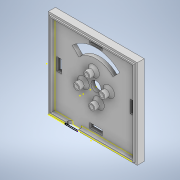
# Autodesk Inventor part: bottomplate
Saved by Autodesk Inventor 2022 (Build 260153000, 153)
## iProperties
Created: 2023-12-05
Part Number: bottomplate
Material: Generisch
Document SubType Name: Modeling
Designer: Marc Panse
Density: 1 g/cm^3
Appearance: Vorgabe
Author: Marc Panse
## iProperties of the stored document bottomplate_3D-Druck.ipt
Created: 2023-12-05
Part Number: bottomplate_3D-Druck
Material: Generisch
Document SubType Name: Modeling
Designer: Marc Panse
Density: 1 g/cm^3
Appearance: Vorgabe
Author: Marc Panse
Autodesk Inventor part; units mm, degrees
ref_plane "YZ Plane" through (0, 0, 0) normal (1, 0, 0) x (0, 1, 0)
ref_plane "XZ Plane" through (0, 0, 0) normal (0, 1, 0) x (-1, 0, 0)
ref_plane "XY Plane" through (0, 0, 0) normal (0, 0, 1) x (1, 0, 0)
sketch "Skizze1" plane through (0, 0, 0) normal (0, 0, 1) x (1, 0, 0)
  line L0 (-33.02, -33.02) -> (33.02, -33.02)
  line L1 (33.02, -33.02) -> (33.02, 33.02)
  line L2 (33.02, 33.02) -> (-33.02, 33.02)
  line L3 (-33.02, 33.02) -> (-33.02, -33.02)
  line L4 (-33.02, -33.02) -> (33.02, 33.02) construction
  line L5 (33.02, -33.02) -> (-33.02, 33.02) construction
  line L6 (-34, -34) -> (34, -34)
  line L7 (34, -34) -> (34, 34)
  line L8 (34, 34) -> (-34, 34)
  line L9 (-34, 34) -> (-34, -34)
  line L10 (-34, -34) -> (34, 34) construction
  line L11 (34, -34) -> (-34, 34) construction
  point P0 (0, 0)
  dimension "d0" = 66.04
  dimension "d1" = 66.04
  dimension "d2" = 68
  dimension "d3" = 68
  constraints: 24 end point, 4 midpoint, 4 parallel, 2 horizontal, 2 perpendicular
  measures "d0" distance of L2.end L1.end
  measures "d1" distance of L1.end L0.end
  measures "d2" distance of L8.end L7.end
  measures "d3" distance of L7.end L6.end
extrude "Extrusion1" add sketch "Skizze1" along normal blind 6.5
sketch "Skizze2" plane through (0, 0, 6.5) normal (0, 0, 1) x (1, 0, 0)
  line L0 (-33.02, 33.02) -> (33.02, 33.02) projected
  line L1 (-33.02, -33.02) -> (33.02, -33.02)
  line L2 (33.02, -33.02) -> (33.02, 33.02)
  line L3 (33.02, 33.02) -> (-33.02, 33.02)
  line L4 (-33.02, 33.02) -> (-33.02, -33.02)
  line L5 (-33.02, -33.02) -> (33.02, 33.02) construction
  line L6 (33.02, -33.02) -> (-33.02, 33.02) construction
  line L7 (34, -34) -> (34, 34) projected
  line L8 (34, 34) -> (-34, 34) projected
  line L9 (-34, 34) -> (-34, -34) projected
  line L10 (-34, -34) -> (34, -34) projected
  line L11 (-33.02, -33.02) -> (-33.02, 33.02) projected
  line L12 (-33.02, 33.02) -> (33.02, 33.02) projected
  line L13 (33.02, 33.02) -> (33.02, -33.02) projected
  line L14 (33.02, -33.02) -> (-33.02, -33.02) projected
  point P0 (0, 0)
  constraints: 12 end point, 2 midpoint, 2 parallel, 1 horizontal, 1 perpendicular
extrude "Extrusion2" add sketch "Skizze2" along normal blind 2 contours L0 L2 L1 L4 | L10 L9 L8 L7
sketch "Skizze3" plane through (0, 0, 6.5) normal (0, 0, -1) x (-1, 0, 0)
  line L0 (-27.94, -27.94) -> (27.94, -27.94)
  line L1 (27.94, -27.94) -> (27.94, 27.94)
  line L2 (27.94, 27.94) -> (-27.94, 27.94)
  line L3 (-27.94, 27.94) -> (-27.94, -27.94)
  line L4 (-27.94, -27.94) -> (27.94, 27.94) construction
  line L5 (27.94, -27.94) -> (-27.94, 27.94) construction
  circle A0 centre (-27.94, 27.94) radius 3.35
  circle A1 centre (27.94, 27.94) radius 3.35
  circle A2 centre (27.94, -27.94) radius 3.35
  circle A3 centre (-27.94, -27.94) radius 3.35
  point P0 (0, 0)
  dimension "d8" = 55.88
  dimension "d9" = 55.88
  dimension "d10" = 6.7
  dimension "d11" = 6.7
  dimension "d12" = 6.7
  dimension "d13" = 6.7
  constraints: 12 end point, 4 centre point, 4 coincident, 2 midpoint, 2 parallel, 1 horizontal, 1 perpendicular
  measures "d8" distance of L2.end L1.end
  measures "d9" distance of L1.end L0.end
  measures "d10" diameter of A0
  measures "d11" diameter of A1
  measures "d12" diameter of A2
  measures "d13" diameter of A3
extrude "Extrusion3" add sketch "Skizze3" along normal blind 5 contours L3 A3 L0 | L0 A3 L3 | A2 L1 L0 | L0 L1 A2 | A0 L2 L3 | L3 L2 A0 | A1 L2 L1 | L1 L2 A1
sketch "Skizze4" plane through (27.94, 27.94, 1.5) normal (0, 0, -1) x (-1, 0, 0)
  circle A0 centre (0, 0) radius 1.1
  circle A1 centre (55.88, 0) radius 3.35 projected
  circle A2 centre (55.88, 0) radius 1.1
  circle A3 centre (55.88, -55.88) radius 3.35 projected
  circle A4 centre (55.88, -55.88) radius 1.1
  circle A5 centre (0, -55.88) radius 3.35 projected
  circle A6 centre (0, -55.88) radius 1.1
  point P0 (27.94, -27.94)
  dimension "d17" = 2.2
  dimension "d18" = 2.2
  dimension "d19" = 2.2
  dimension "d20" = 2.2
  constraints: 4 centre point, 3 coincident
  measures "d17" diameter of A0
  measures "d18" diameter of A2
  measures "d19" diameter of A4
  measures "d20" diameter of A6
extrude "Extrusion4" cut sketch "Skizze4" against normal blind 5 contours A0 | A2 | A4 | A6
sketch "Skizze5" plane through (0, 0, 0) normal (0, 0, -1) x (-1, 0, 0)
  line L0 (-34, -34) -> (-34, 34) projected
  line L1 (34, -34) -> (-34, -34) projected
  line L2 (34, 34) -> (34, -34) projected
  line L3 (-34, 34) -> (34, 34) projected
  line L4 (33.02, -33.02) -> (33.02, 33.02) projected
  line L5 (-33.02, -33.02) -> (33.02, -33.02) projected
  line L6 (-33.02, 33.02) -> (-33.02, -33.02) projected
  line L7 (33.02, 33.02) -> (-33.02, 33.02) projected
  point P0 (0, 0)
extrude "Extrusion5" add sketch "Skizze5" along normal blind 4
sketch "Skizze6" plane through (0, 0, -4) normal (0, 0, -1) x (-1, 0, 0)
  line L0 (-33.02, -33.02) -> (33.02, -33.02)
  line L1 (33.02, -33.02) -> (33.02, 33.02)
  line L2 (33.02, 33.02) -> (-33.02, 33.02)
  line L3 (-33.02, 33.02) -> (-33.02, -33.02)
  line L4 (-33.02, -33.02) -> (33.02, 33.02) construction
  line L5 (33.02, -33.02) -> (-33.02, 33.02) construction
  line L6 (33.02, -33.02) -> (20.02, -33.02)
  line L7 (-33.02, -33.02) -> (33.02, -33.02) projected
  line L8 (20.02, -33.02) -> (10.08, -33.02)
  line L9 (34, -34) -> (-34, -34) projected
  line L10 (10.08, -33.02) -> (20.02, -33.02)
  line L11 (20.02, -33.02) -> (20.02, -34)
  line L12 (20.02, -34) -> (10.08, -34)
  line L13 (10.08, -34) -> (10.08, -33.02)
  point P0 (0, 0)
  point P1 (-24.13, -33.02)
  point P2 (24.13, -33.02)
  dimension "d25" = 66.04
  dimension "d26" = 66.04
  dimension "d27" = 13
  dimension "d28" = 9.94
  constraints: 24 end point, 4 parallel, 3 point on line, 2 horizontal, 2 midpoint, 2 perpendicular
  measures "d25" distance of L2.end L1.end
  measures "d26" distance of L1.end L0.end
  measures "d27" distance of L0.end L6.end
  measures "d28" distance of L6.end L8.end
extrude "Extrusion6" cut sketch "Skizze6" against normal blind 4 contours L0 L11 L9 L13
fillet "Rundung2" radius 1.75 2 edges at (-10.08, -33.51, 0) (-20.02, -33.51, 0)
sketch "Skizze7" plane through (0, 0, -4) normal (0, 0, -1) x (-1, 0, 0)
  line L0 (34, 34) -> (-34, 34) projected
  line L1 (-34, -34) -> (34, -34)
  line L2 (34, -34) -> (34, 34)
  line L3 (34, 34) -> (-34, 34)
  line L4 (-34, 34) -> (-34, -34)
  line L5 (-34, -34) -> (34, 34) construction
  line L6 (34, -34) -> (-34, 34) construction
  line L7 (-35, -35) -> (35, -35)
  line L8 (35, -35) -> (35, 35)
  line L9 (35, 35) -> (-35, 35)
  line L10 (-35, 35) -> (-35, -35)
  line L11 (-35, -35) -> (35, 35) construction
  line L12 (35, -35) -> (-35, 35) construction
  point P0 (0, 0)
  point P1 (-34, 34)
  dimension "d32" = 70
  dimension "d33" = 70
  constraints: 24 end point, 4 midpoint, 4 parallel, 2 horizontal, 2 perpendicular
  measures "d32" distance of L9.end L8.end
  measures "d33" distance of L8.end L7.end
extrude "Extrusion7" add sketch "Skizze7" against normal up to surface (12.5 mm away)
sketch "Skizze8" plane through (-20.02, -34, -4) normal (0, 1, 0) x (1, 0, 0)
  line L0 (9.94, -2.25) -> (9.94, 0) projected
  line L1 (0, 0) -> (9.94, 0) projected
  line L2 (0, 0) -> (0, -2.25) projected
  arc A0 (0, -2.25) -> (1.75, -4) centre (1.75, -2.25) ccw projected
  line L3 (1.75, -4) -> (8.19, -4) projected
  arc A1 (8.19, -4) -> (9.94, -2.25) centre (8.19, -2.25) ccw projected
  point P0 (20.02, -4)
extrude "Extrusion8" cut sketch "Skizze8" against normal blind 10
sketch "Skizze9" plane through (0, 0, -4) normal (0, 0, -1) x (-1, 0, 0)
  line L0 (-33.52, 33.52) -> (33.52, 33.52)
  line L1 (33.52, 33.52) -> (33.52, -33.52)
  line L2 (33.52, -33.52) -> (-33.52, -33.52)
  line L3 (-33.52, -33.52) -> (-33.52, 33.52)
  line L4 (-33.52, 33.52) -> (33.52, -33.52) construction
  line L5 (33.52, 33.52) -> (-33.52, -33.52) construction
  line L6 (10.08, -35) -> (10.08, -33.02) projected
  line L7 (10.08, -33.02) -> (-33.02, -33.02) projected
  line L8 (-33.02, -33.02) -> (-33.02, 33.02) projected
  line L9 (-33.02, 33.02) -> (33.02, 33.02) projected
  line L10 (33.02, 33.02) -> (33.02, -33.02) projected
  line L11 (33.02, -33.02) -> (20.02, -33.02) projected
  line L12 (20.02, -33.02) -> (20.02, -35) projected
  line L13 (20.02, -35) -> (35, -35) projected
  line L14 (35, -35) -> (35, 35) projected
  line L15 (35, 35) -> (-35, 35) projected
  line L16 (-35, 35) -> (-35, -35) projected
  line L17 (-35, -35) -> (10.08, -35) projected
  point P0 (0, 0)
  point P1 (10.08, -33.52)
  point P2 (20.02, -33.52)
  dimension "d38" = 67.04
  dimension "d39" = 67.04
  constraints: 12 end point, 2 midpoint, 2 parallel, 1 horizontal, 1 perpendicular
  measures "d38" distance of L1.end L2.end
  measures "d39" distance of L0.end L1.end
extrude "Extrusion9" cut sketch "Skizze9" against normal up to surface (10.5 mm away) contours L0 L1 L2 L12 L11 L10 L9 L8 L7 L6 L3
fillet "Rundung3" radius 2 4 edges at (31.29, -27.94, 6.5) (31.29, 27.94, 6.5) (-24.59, 27.94, 6.5) (-24.59, -27.94, 6.5)
sketch "Skizze10" plane through (-35, -35, -4) normal (-1, 0, 0) x (0, 0, 1)
  point P0 (4, 35)
sketch "Skizze11" plane through (0, 0, 8.5) normal (0, 0, 1) x (1, 0, 0)
  point P0 (0, 0)
sketch "Skizze12" plane through (-18.27, -33.02, 0) normal (0, 1, 0) x (1, 0, 0)
  line L0 (-1.75, 1.75) -> (-1.75, -6.5) projected
  line L1 (8.19, -6.5) -> (-1.75, -6.5) projected
  line L2 (8.19, -6.5) -> (8.19, 1.75) projected
  arc A0 (6.44, 0) -> (8.19, 1.75) centre (6.44, 1.75) ccw projected
  line L3 (6.44, 0) -> (0, 0) projected
  arc A1 (-1.75, 1.75) -> (0, 0) centre (0, 1.75) ccw projected
  point P0 (18.27, 0)
extrude "Extrusion10" cut sketch "Skizze12" against normal up to surface (0.5 mm away)
sketch "Skizze13" plane through (0, 0, -4) normal (0, 0, -1) x (-1, 0, 0)
  circle A0 centre (0, 0) radius 4
  line L0 (0, 0) -> (-10.0581, 1.7135)
  line L1 (0, 0) -> (10.203, 0) construction
  line L2 (0, 0) -> (1.8539, 9.7483)
  line L3 (0, 0) -> (9.923, 0) construction
  line L4 (0, 0) -> (9.888, -2.1637)
  line L5 (0, 0) -> (10.122, 0) construction
  line L6 (0, 0) -> (-2.0234, -10.1982)
  line L7 (0, 0) -> (10.397, 0) construction
  circle A1 centre (-2.0234, -10.1982) radius 2.5
  circle A2 centre (-10.0581, 1.7135) radius 2.5
  circle A3 centre (1.8539, 9.7483) radius 2.5
  circle A4 centre (9.888, -2.1637) radius 2.5
  dimension "d59" = 8
  dimension "d60" = 10.203
  dimension "d61" = 170.332
  dimension "d62" = 9.923
  dimension "d63" = 79.232
  dimension "d64" = 10.122
  dimension "d65" = 12.343
  dimension "d66" = 10.397
  dimension "d67" = 101.222
  dimension "d68" = 5
  dimension "d69" = 5
  dimension "d70" = 5
  dimension "d71" = 5
  constraints: 16 end point, 5 centre point, 5 coincident, 4 equal length, 4 horizontal
  measures "d59" diameter of A0
  measures "d60" distance of L0.start L0.end
  measures "d61" angle of L1 L0
  measures "d62" distance of L0.start L2.end
  measures "d63" angle of L3 L2
  measures "d64" distance of L0.start L4.end
  measures "d65" angle of L4 L5
  measures "d66" distance of L0.start L6.end
  measures "d67" angle of L6 L7
  measures "d68" diameter of A1
  measures "d69" diameter of A2
  measures "d70" diameter of A3
  measures "d71" diameter of A4
extrude "Extrusion11" add sketch "Skizze13" against normal up to surface (10.5 mm away) contours A1 | A2 | A3 | A4
sketch "Skizze14" plane through (-9.888, -2.1637, -4) normal (0, 0, -1) x (-1, 0, 0)
  circle A0 centre (0, 0) radius 2.5 projected
  circle A1 centre (-11.9114, -8.0345) radius 2.5 projected
  circle A2 centre (-19.9461, 3.8772) radius 2.5 projected
  circle A3 centre (-8.0341, 11.912) radius 2.5 projected
  point P0 (-9.888, 2.1637)
extrude "Extrusion12" cut sketch "Skizze14" against normal blind 5.5
fillet "Rundung4" radius 4 4 edges at (12.5581, 1.7135, 6.5) (0.6461, 9.7483, 6.5) (-7.388, -2.1637, 6.5) (4.5234, -10.1982, 6.5)
sketch "Skizze15" plane through (-9.888, -2.1637, 1.5) normal (0, 0, -1) x (-1, 0, 0)
  circle A0 centre (0, 0) radius 1
  circle A1 centre (-11.9114, -8.0345) radius 2.5 projected
  circle A2 centre (-11.9114, -8.0345) radius 1
  circle A3 centre (-19.9461, 3.8772) radius 2.5 projected
  circle A4 centre (-19.9461, 3.8772) radius 1
  circle A5 centre (-8.0341, 11.912) radius 2.5 projected
  circle A6 centre (-8.0341, 11.912) radius 1
  point P0 (-9.888, 2.1637)
  dimension "d77" = 2
  dimension "d78" = 2
  dimension "d79" = 2
  dimension "d80" = 2
  constraints: 4 centre point, 3 coincident
  measures "d77" diameter of A0
  measures "d78" diameter of A2
  measures "d79" diameter of A4
  measures "d80" diameter of A6
extrude "Extrusion13" cut sketch "Skizze15" against normal blind 5 contours A0 | A2 | A4 | A6
chamfer "Fase1" distance 4 angle 45 4 edges at (-33.52, 0, 6.5) (0, -33.52, 6.5) (0, 33.52, 6.5) (33.52, 0, 6.5)
sketch "Skizze16" plane through (10.0581, 1.7135, 1.5) normal (0, 0, -1) x (-1, 0, 0)
  circle A0 centre (0, 0) radius 1.6
  circle A1 centre (8.0347, -11.9117) radius 1 projected
  circle A2 centre (8.0347, -11.9117) radius 1.6
  circle A3 centre (11.912, 8.0348) radius 1 projected
  circle A4 centre (11.912, 8.0348) radius 1.6
  circle A5 centre (19.9461, -3.8772) radius 1 projected
  circle A6 centre (19.9461, -3.8772) radius 1.6
  point P0 (10.0581, -1.7135)
  dimension "d86" = 3.2
  dimension "d87" = 3.2
  dimension "d88" = 3.2
  dimension "d89" = 3.2
  constraints: 4 centre point, 3 coincident
  measures "d86" diameter of A0
  measures "d87" diameter of A2
  measures "d88" diameter of A4
  measures "d89" diameter of A6
extrude "Extrusion14" cut sketch "Skizze16" against normal blind 10 contours A0 | A1 | A2 | A3 | A4 | A5 | A6
chamfer "Fase2" distance 2 angle 45 4 edges at (-8.288, -2.1637, 8.5) (3.6234, -10.1982, 8.5) (11.6581, 1.7135, 8.5) (-0.2539, 9.7483, 8.5)
sketch "Skizze17" plane through (0, 0, 8.5) normal (0, 0, 1) x (1, 0, 0)
  circle A0 centre (10.0581, 1.7135) radius 3.6 projected
  circle A1 centre (-9.888, -2.1637) radius 3.6 projected
  line L0 (35, 35) -> (-35, 35) projected
  line L1 (-35, 35) -> (-35, -35) projected
  line L2 (-35, -35) -> (35, -35) projected
  line L3 (35, -35) -> (35, 35) projected
  circle A2 centre (2.0234, -10.1982) radius 3.6 projected
  circle A3 centre (-1.8539, 9.7483) radius 3.6 projected
  line L4 (-35, -35) -> (35, -35) projected
  line L5 (-35, 35) -> (35, 35)
  line L6 (35, 35) -> (35, -35)
  line L7 (35, -35) -> (-35, -35)
  line L8 (-35, -35) -> (-35, 35)
  point P0 (0, 0)
  constraints: 8 end point, 2 parallel, 1 horizontal, 1 perpendicular
extrude "Extrusion15" cut sketch "Skizze17" against normal blind 10
sketch "Skizze18" plane through (-9.888, -2.1637, 1.5) normal (0, 0, -1) x (-1, 0, 0)
  line L0 (7.2248, 22.465) -> (-25.8707, 22.465)
  line L1 (-25.8707, 22.465) -> (-25.8707, -11.357)
  line L2 (-25.8707, -11.357) -> (7.2248, -11.357)
  line L3 (7.2248, -11.357) -> (7.2248, 22.465)
  line L4 (6.4983, 16.5724) -> (-29.7453, 16.5724)
  line L5 (-29.7453, 16.5724) -> (-29.7453, -17.4918)
  line L6 (-29.7453, -17.4918) -> (6.4983, -17.4918)
  line L7 (6.4983, -17.4918) -> (6.4983, 16.5724)
  point P0 (-9.888, 2.1637)
  point P1 (-25.8707, 16.5724)
  point P2 (6.4983, -11.357)
  constraints: 16 end point, 4 parallel, 2 horizontal, 2 perpendicular
extrude "Extrusion16" cut sketch "Skizze18" against normal blind 10
sketch "Skizze19" plane through (0, 0, -4) normal (0, 0, -1) x (-1, 0, 0)
  line L0 (33.52, -33.52) -> (20.02, -33.52) projected
  line L1 (20.02, -33.52) -> (20.02, -35) projected
  line L2 (20.02, -35) -> (35, -35) projected
  line L3 (35, -35) -> (35, 35) projected
  line L4 (35, 35) -> (-35, 35) projected
  line L5 (-35, 35) -> (-35, -35) projected
  line L6 (-35, -35) -> (10.08, -35) projected
  line L7 (10.08, -35) -> (10.08, -33.52) projected
  line L8 (10.08, -33.52) -> (-33.52, -33.52) projected
  line L9 (-33.52, -33.52) -> (-33.52, 33.52) projected
  line L10 (-33.52, 33.52) -> (33.52, 33.52) projected
  line L11 (33.52, 33.52) -> (33.52, -33.52) projected
  line L12 (-33.52, 33.52) -> (33.52, 33.52) projected
  line L13 (33.52, 33.52) -> (33.52, -33.52) projected
  line L14 (-33.52, 33.52) -> (33.52, 33.52)
  line L15 (33.52, 33.52) -> (33.52, -33.52)
  line L16 (33.52, -33.52) -> (-33.52, -33.52)
  line L17 (-33.52, -33.52) -> (-33.52, 33.52)
  line L18 (-35, 35) -> (-35, -35) projected
  line L19 (35, -35) -> (35, 35) projected
  line L20 (-35, 35) -> (35, 35)
  line L21 (35, 35) -> (35, -35)
  line L22 (35, -35) -> (-35, -35)
  line L23 (-35, -35) -> (-35, 35)
  point P0 (0, 0)
  point P1 (10.08, -35)
  constraints: 16 end point, 4 parallel, 2 horizontal, 2 perpendicular
extrude "Extrusion17" add sketch "Skizze19" along normal blind 3
fillet "Rundung5" radius 1.75 2 edges at (-10.08, -34.26, -4) (-20.02, -34.26, -4)
sketch "Skizze20" plane through (-10.0979, -35, -1.5) normal (0, -1, 0) x (1, 0, 0)
  point P0 (10.0979, 1.5)
sketch "Skizze21" plane through (0, 0, -1.5) normal (0, 0, 1) x (1, 0, 0)
  line L0 (-10.0979, -33.52) -> (33.52, -33.52) projected
  line L1 (-33.52, 33.52) -> (-33.52, -33.52) projected
  line L2 (33.52, -33.52) -> (-33.52, -33.52)
  line L3 (-33.52, -33.52) -> (-33.52, 33.52)
  line L4 (-33.52, 33.52) -> (33.52, 33.52)
  line L5 (33.52, 33.52) -> (33.52, -33.52)
  line L6 (32.52, 32.52) -> (-32.52, 32.52)
  line L7 (-32.52, 32.52) -> (-32.52, -32.52)
  line L8 (-32.52, -32.52) -> (32.52, -32.52)
  line L9 (32.52, -32.52) -> (32.52, 32.52)
  line L10 (32.52, 32.52) -> (-32.52, -32.52) construction
  line L11 (-32.52, 32.52) -> (32.52, -32.52) construction
  point P0 (0, 0)
  dimension "d102" = 65.04
  dimension "d103" = 65.04
  constraints: 20 end point, 4 parallel, 2 horizontal, 2 midpoint, 2 perpendicular
  measures "d102" distance of L8.end L7.end
  measures "d103" distance of L7.end L6.end
extrude "Extrusion18" add sketch "Skizze21" along normal blind 2 and the other way blind 3
sketch "Skizze22" plane through (0, 0, 0.5) normal (0, 0, 1) x (1, 0, 0)
  line L0 (-33.52, -33.52) -> (-20.0021, -33.52) projected
  line L1 (-32.52, -32.52) -> (32.52, -32.52) projected
  line L2 (-20.0021, -33.52) -> (-10.0737, -33.52)
  line L3 (-10.0737, -33.52) -> (-10.0737, -32.52)
  line L4 (-10.0737, -32.52) -> (-20.0021, -32.52)
  line L5 (-20.0021, -32.52) -> (-20.0021, -33.52)
  point P0 (0, 0)
  constraints: 8 end point, 2 parallel, 1 horizontal, 1 perpendicular, 1 point on line
sketch "Skizze23" plane through (-10.0979, -33.52, -1.5) normal (0, -1, 0) x (1, 0, 0)
  line L0 (-23.4221, 0) -> (-9.9041, 0) projected
  arc A0 (-9.9041, 0) -> (-9.9221, -0.25) centre (-8.1721, -0.25) ccw projected
  line L1 (-9.9221, -0.75) -> (-9.9221, -0.25) projected
  arc A1 (-9.9221, -0.75) -> (-8.1721, -2.5) centre (-8.1721, -0.75) ccw projected
  line L2 (-1.7321, -2.5) -> (-8.1721, -2.5) projected
  arc A2 (-1.7321, -2.5) -> (0.0179, -0.75) centre (-1.7321, -0.75) ccw projected
  line L3 (0.0179, -0.25) -> (0.0179, -0.75) projected
  arc A3 (0.0179, -0.25) -> (0, 0) centre (-1.7321, -0.25) ccw projected
  line L4 (0, 0) -> (43.6179, 0) projected
  line L5 (43.6179, 0) -> (43.6179, 2) projected
  line L6 (-23.4221, 2) -> (43.6179, 2) projected
  line L7 (-23.4221, 0) -> (-23.4221, 2) projected
  line L8 (-22.4221, 2) -> (42.6179, 2) projected
  line L9 (-9.9041, 0) -> (0, 0)
  line L10 (0, 0) -> (0, 2)
  line L11 (0, 2) -> (-9.9041, 2)
  line L12 (-9.9041, 2) -> (-9.9041, 0)
  point P0 (10.0979, 1.5)
  constraints: 8 end point, 2 parallel, 1 horizontal, 1 perpendicular, 1 point on line
extrude "Extrusion19" cut sketch "Skizze23" against normal blind 10 contours L9 A3 L3 A2 L2 A1 L1 A0 | L12 L6 L10 L9
sketch "Skizze24" plane through (0, 0, -4) normal (0, 0, 1) x (1, 0, 0)
  circle A0 centre (0, 0) radius 4
  line L0 (0, 0) -> (-10.0581, 1.7135)
  line L1 (0, 0) -> (10.203, 0) construction
  line L2 (0, 0) -> (1.8539, 9.7483)
  line L3 (0, 0) -> (9.923, 0) construction
  line L4 (0, 0) -> (9.888, -2.1637)
  line L5 (0, 0) -> (10.122, 0) construction
  line L6 (0, 0) -> (-2.0234, -10.1982)
  line L7 (0, 0) -> (10.397, 0) construction
  circle A1 centre (-2.0234, -10.1982) radius 2.5
  circle A2 centre (-10.0581, 1.7135) radius 2.5
  circle A3 centre (1.8539, 9.7483) radius 2.5
  circle A4 centre (9.888, -2.1637) radius 2.5
  dimension "d110" = 8
  dimension "d111" = 10.203
  dimension "d112" = 170.332
  dimension "d113" = 9.923
  dimension "d114" = 79.232
  dimension "d115" = 10.122
  dimension "d116" = 12.343
  dimension "d117" = 10.397
  dimension "d118" = 101.222
  dimension "d119" = 5
  dimension "d120" = 5
  dimension "d121" = 5
  dimension "d122" = 5
  constraints: 16 end point, 5 centre point, 5 coincident, 4 equal length, 4 horizontal
  measures "d110" diameter of A0
  measures "d111" distance of L6.start L0.end
  measures "d112" angle of L1 L0
  measures "d113" distance of L6.start L2.end
  measures "d114" angle of L3 L2
  measures "d115" distance of L6.start L4.end
  measures "d116" angle of L4 L5
  measures "d117" distance of L6.start L6.end
  measures "d118" angle of L6 L7
  measures "d119" diameter of A1
  measures "d120" diameter of A2
  measures "d121" diameter of A3
  measures "d122" diameter of A4
extrude "Extrusion20" add sketch "Skizze24" along normal blind 10 contours A1 | A2 | A3 | A4
mirror "Spiegeln1" about plane through (0, 0, 0) normal (1, 0, 0) of "Extrusion20"
sketch "Skizze25" plane through (0, 0, 6) normal (0, 0, 1) x (1, 0, 0)
  point P0 (0, 0)
sketch "Skizze26" plane through (0, 0, 6) normal (0, 0, 1) x (1, 0, 0)
  arc A0 (0, 8.0711) -> (0, 11.4254) centre (1.8539, 9.7483) ccw projected
  arc A1 (0, 11.4254) -> (0, 8.0711) centre (-1.8539, 9.7483) ccw projected
  arc A2 (-8.3983, -0.156) -> (-11.5478, -0.2942) centre (-10.0581, 1.7135) ccw projected
  arc A3 (-11.5478, -0.2942) -> (-8.3983, -0.156) centre (-9.888, -2.1637) ccw projected
  arc A4 (0, -8.7299) -> (0, -11.6665) centre (-2.0234, -10.1982) ccw projected
  arc A5 (0, -11.6665) -> (0, -8.7299) centre (2.0234, -10.1982) ccw projected
  arc A6 (8.3983, -0.156) -> (11.5478, -0.2942) centre (9.888, -2.1637) ccw projected
  arc A7 (11.5478, -0.2942) -> (8.3983, -0.156) centre (10.0581, 1.7135) ccw projected
  arc A8 (0, 8.0711) -> (0, 11.4254) centre (1.8539, 9.7483) ccw projected
  circle A9 centre (1.8539, 9.7483) radius 2.5
  circle A10 centre (-10.0581, 1.7135) radius 2.5
  circle A11 centre (9.888, -2.1637) radius 2.5
  circle A12 centre (-2.0234, -10.1982) radius 2.5
  circle A13 centre (2.0234, -10.1982) radius 2.5
  circle A14 centre (10.0581, 1.7135) radius 2.5
  circle A15 centre (-1.8539, 9.7483) radius 2.5
  circle A16 centre (-9.888, -2.1637) radius 2.5
  point P0 (0, 0)
  point P1 (11.5478, -0.2942)
  point P2 (8.3983, -0.156)
  point P3 (0, -11.6665)
  point P4 (0, 11.4254)
  point P5 (-11.5478, -0.2942)
  point P6 (-8.3983, -0.156)
  constraints: 8 centre point, 8 coincident
extrude "Extrusion21" cut sketch "Skizze26" against normal blind 10 contours A15 A0 | A16 A2 | A13 A4 | A14 A6
sketch "Skizze27" plane through (-1.8539, 9.7483, 6) normal (0, 0, 1) x (1, 0, 0)
  circle A0 centre (0, 0) radius 2.5 projected
  circle A1 centre (0, 0) radius 1.6
  circle A2 centre (-8.0341, -11.912) radius 2.5 projected
  circle A3 centre (-8.0341, -11.912) radius 1.6
  circle A4 centre (11.912, -8.0348) radius 2.5 projected
  circle A5 centre (11.912, -8.0348) radius 1.6
  circle A6 centre (3.8773, -19.9465) radius 2.5 projected
  circle A7 centre (3.8773, -19.9465) radius 1.6
  point P0 (1.8539, -9.7483)
  dimension "d127" = 3.2
  dimension "d128" = 3.2
  dimension "d129" = 3.2
  dimension "d130" = 3.2
  constraints: 4 centre point, 4 coincident
  measures "d127" diameter of A1
  measures "d128" diameter of A3
  measures "d129" diameter of A5
  measures "d130" diameter of A7
extrude "Extrusion22" cut sketch "Skizze27" against normal blind 20 contours A1 | A3 | A5 | A7
sketch "Skizze28" plane through (0, 0, -4) normal (0, 0, 1) x (1, 0, 0)
  line L0 (-18.27, -35) -> (-18.27, -32.52) projected
  line L1 (-11.83, -35) -> (-18.27, -35) projected
  line L2 (-11.83, -35) -> (-11.83, -32.52) projected
  line L3 (-11.83, -32.52) -> (32.52, -32.52) projected
  line L4 (32.52, -32.52) -> (32.52, 32.52) projected
  line L5 (32.52, 32.52) -> (-32.52, 32.52) projected
  line L6 (-32.52, 32.52) -> (-32.52, -32.52) projected
  line L7 (-32.52, -32.52) -> (-18.27, -32.52) projected
  circle A0 centre (-9.888, -2.1637) radius 2.5 projected
  circle A1 centre (10.0581, 1.7135) radius 2.5 projected
  circle A2 centre (2.0234, -10.1982) radius 2.5 projected
  circle A3 centre (-1.8539, 9.7483) radius 2.5 projected
  point P0 (0, 0)
sketch "Skizze29" plane through (0, 0, 0.5) normal (0, 0, 1) x (1, 0, 0)
  line L0 (-10.0979, -32.52) -> (-10.0979, -33.52) projected
  line L1 (-10.0979, -33.52) -> (33.52, -33.52) projected
  line L2 (33.52, -33.52) -> (33.52, 33.52) projected
  line L3 (33.52, 33.52) -> (-33.52, 33.52) projected
  line L4 (-33.52, 33.52) -> (-33.52, -33.52) projected
  line L5 (-33.52, -33.52) -> (-20.0021, -33.52) projected
  line L6 (-20.0021, -33.52) -> (-20.0021, -32.52) projected
  line L7 (-20.0021, -32.52) -> (-32.52, -32.52) projected
  line L8 (-32.52, -32.52) -> (-32.52, 32.52) projected
  line L9 (-32.52, 32.52) -> (32.52, 32.52) projected
  line L10 (32.52, 32.52) -> (32.52, -32.52) projected
  line L11 (32.52, -32.52) -> (-10.0979, -32.52) projected
  point P0 (0, 0)
extrude "Extrusion23" cut sketch "Skizze29" against normal blind 1
sketch "Skizze30" plane through (0, 0, -4) normal (0, 0, 1) x (1, 0, 0)
  circle A0 centre (0, 0) radius 4
  dimension "d135" = 8
  constraints: 1 centre point, 1 coincident
  measures "d135" diameter of A0
extrude "Extrusion24" cut sketch "Skizze30" against normal blind 10
sketch "Skizze31" plane through (-9.888, -2.1637, 6) normal (0, 0, 1) x (1, 0, 0)
  circle A0 centre (8.0341, 11.912) radius 2.5 projected
  circle A1 centre (8.0341, 11.912) radius 1.6 projected
  circle A2 centre (8.0341, 11.912) radius 2.5 projected
  circle A3 centre (0, 0) radius 1.6 projected
  circle A4 centre (0, 0) radius 2.5 projected
  circle A5 centre (11.9114, -8.0345) radius 1.6 projected
  circle A6 centre (11.9114, -8.0345) radius 2.5 projected
  circle A7 centre (19.9461, 3.8772) radius 1.6 projected
  circle A8 centre (19.9461, 3.8772) radius 2.5 projected
  point P0 (9.888, 2.1637)
extrude "Extrusion25" cut sketch "Skizze31" against normal blind 4.5
fillet "Rundung6" radius 2 8 edges at (-9.7785, -4.6613, -4) (-9.9976, 0.3339, -4) (4.5234, -10.1982, -4) (-0.4766, -10.1982, -4) (10.1676, 4.2111, -4) (9.9485, -0.7841, -4) (-4.3539, 9.7483, -4) (0.6461, 9.7483, -4)
sketch "Skizze32" plane through (-1.8539, 9.7483, 1.5) normal (0, 0, 1) x (1, 0, 0)
  line L0 (-27.1461, -38.7483) -> (30.8539, -38.7483)
  line L1 (30.8539, -38.7483) -> (30.8539, 19.2517)
  line L2 (30.8539, 19.2517) -> (-27.1461, 19.2517)
  line L3 (-27.1461, 19.2517) -> (-27.1461, -38.7483)
  line L4 (-27.1461, -38.7483) -> (30.8539, 19.2517) construction
  line L5 (30.8539, -38.7483) -> (-27.1461, 19.2517) construction
  line L6 (-25.1461, -14.7483) -> (-29.1461, -14.7483)
  line L7 (-29.1461, -14.7483) -> (-29.1461, -4.7483)
  line L8 (-29.1461, -4.7483) -> (-25.1461, -4.7483)
  line L9 (-25.1461, -4.7483) -> (-25.1461, -14.7483)
  line L10 (-25.1461, -14.7483) -> (-29.1461, -4.7483) construction
  line L11 (-29.1461, -14.7483) -> (-25.1461, -4.7483) construction
  line L12 (6.8539, 21.2517) -> (-3.1461, 21.2517)
  line L13 (-3.1461, 21.2517) -> (-3.1461, 17.2517)
  line L14 (-3.1461, 17.2517) -> (6.8539, 17.2517)
  line L15 (6.8539, 17.2517) -> (6.8539, 21.2517)
  line L16 (6.8539, 21.2517) -> (-3.1461, 17.2517) construction
  line L17 (-3.1461, 21.2517) -> (6.8539, 17.2517) construction
  line L18 (32.8539, -14.7483) -> (28.8539, -14.7483)
  line L19 (28.8539, -14.7483) -> (28.8539, -4.7483)
  line L20 (28.8539, -4.7483) -> (32.8539, -4.7483)
  line L21 (32.8539, -4.7483) -> (32.8539, -14.7483)
  line L22 (32.8539, -14.7483) -> (28.8539, -4.7483) construction
  line L23 (28.8539, -14.7483) -> (32.8539, -4.7483) construction
  line L24 (6.8539, -40.7483) -> (-3.1461, -40.7483)
  line L25 (-3.1461, -40.7483) -> (-3.1461, -36.7483)
  line L26 (-3.1461, -36.7483) -> (6.8539, -36.7483)
  line L27 (6.8539, -36.7483) -> (6.8539, -40.7483)
  line L28 (6.8539, -40.7483) -> (-3.1461, -36.7483) construction
  line L29 (-3.1461, -40.7483) -> (6.8539, -36.7483) construction
  point P0 (1.8539, -9.7483)
  point P1 (-27.1461, -9.7483)
  point P2 (1.8539, 19.2517)
  point P3 (30.8539, -9.7483)
  point P4 (1.8539, -38.7483)
  dimension "d141" = 58
  dimension "d142" = 58
  dimension "d143" = 4
  dimension "d144" = 10
  dimension "d145" = 10
  dimension "d146" = 4
  dimension "d147" = 4
  dimension "d148" = 10
  dimension "d149" = 10
  dimension "d150" = 4
  constraints: 60 end point, 14 midpoint, 10 parallel, 5 horizontal, 5 perpendicular
  measures "d141" distance of L2.end L1.end
  measures "d142" distance of L1.end L0.end
  measures "d143" distance of L7.end L8.end
  measures "d144" distance of L6.end L7.end
  measures "d145" distance of L14.end L13.end
  measures "d146" distance of L13.end L12.end
  measures "d147" distance of L19.end L20.end
  measures "d148" distance of L18.end L19.end
  measures "d149" distance of L25.end L26.end
  measures "d150" distance of L24.end L25.end
extrude "Extrusion26" cut sketch "Skizze32" against normal blind 20 contours L25 L26 L27 L0 | L0 L27 L24 L25 | L6 L7 L8 L3 | L3 L8 L9 L6 | L18 L19 L20 L1 | L1 L20 L21 L18 | L13 L12 L15 L2 | L2 L15 L14 L13
sketch "Skizze33" plane through (0, 0, -4) normal (0, 0, 1) x (1, 0, 0)
  circle A0 centre (0, 0) radius 23.2
  circle A1 centre (0, 0) radius 19
  circle A2 centre (0, 0) radius 4 projected
  circle A3 centre (0, 0) radius 26.5
  line L0 (0, 0) -> (-22.8248, 22.8248)
  line L1 (0, 0) -> (32.2792, 0) construction
  line L2 (0, 0) -> (20.7835, 20.7835)
  line L3 (0, 0) -> (29.3923, 0) construction
  point P0 (18.7383, 18.7383)
  point P1 (-18.7383, 18.7383)
  point P2 (-13.435, 13.435)
  point P3 (13.435, 13.435)
  dimension "d153" = 46.4
  dimension "d154" = 38
  dimension "d155" = 53
  dimension "d156" = 135
  dimension "d157" = 45
  constraints: 8 end point, 3 centre point, 3 coincident, 2 equal length, 2 horizontal
  measures "d153" diameter of A0
  measures "d154" diameter of A1
  measures "d155" diameter of A3
  measures "d156" angle of L1 L0
  measures "d157" angle of L3 L2
extrude "Extrusion27" cut sketch "Skizze33" against normal blind 20 contours L2 A1 L0 A0 | A0 L0 A3 L2 picked at (4.1291, 21.2776) picked at (-15.0601, 20.2735)
